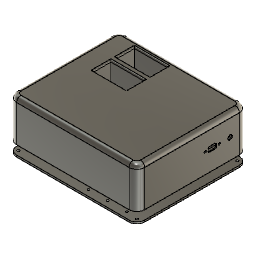
synth case (Autodesk Fusion 360 design; units mm, degrees)
Autodesk Fusion 360 part; units mm, degrees
note: some values were not read from the file. Set by a fixed rule: which sketch regions a step uses.
(part 1 of 2)
sketch "Sketch1" plane through (0, 0, 0) normal (0, 0, 1) x (1, 0, 0) in component "Lid"
  line L0 (6, 0) -> (164, 0) construction
  line L1 (170, 6) -> (170, 139) construction
  line L2 (164, 145) -> (6, 145) construction
  line L3 (0, 139) -> (0, 6) construction
  line L4 (0, 145) -> (10, 145) construction
  line L5 (10, 145) -> (10, 129) construction
  line L6 (10, 129) -> (0, 129) construction
  line L7 (0, 129) -> (0, 145) construction
  line L8 (10, 129) -> (90, 129)
  line L9 (90, 129) -> (90, 126)
  line L10 (90, 126) -> (10, 126)
  line L11 (10, 126) -> (10, 129)
  line L12 (10, 126) -> (10, 96) construction
  line L13 (10, 96) -> (90, 96)
  line L14 (90, 96) -> (90, 93)
  line L15 (90, 93) -> (10, 93)
  line L16 (10, 93) -> (10, 96)
  circle A0 centre (98.5, 65.3144) radius 3.75
  line L17 (24, 66.323) -> (31, 66.323)
  line L18 (33, 64.323) -> (33, 57.323)
  line L19 (31, 55.323) -> (24, 55.323)
  line L20 (22, 57.323) -> (22, 64.323)
  arc A1 (33, 64.323) -> (31, 66.323) centre (31, 64.323) ccw
  arc A2 (31, 55.323) -> (33, 57.323) centre (31, 57.323) ccw
  arc A3 (24, 66.323) -> (22, 64.323) centre (24, 64.323) ccw
  arc A4 (22, 57.323) -> (24, 55.323) centre (24, 57.323) ccw
  line L21 (50, 93) -> (50, 0) construction
  line L22 (98.5, 65.3144) -> (98.5, 57.5144) construction
  circle A5 centre (98.5, 57.5144) radius 1.45
  circle A6 centre (125.5, 65.3144) radius 3.75
  circle A7 centre (125.5, 57.5144) radius 1.45
  circle A8 centre (152.5, 65.3144) radius 3.75
  circle A9 centre (152.5, 57.5144) radius 1.45
  circle A10 centre (98.5, 38.3144) radius 3.75
  circle A11 centre (98.5, 30.5144) radius 1.45
  circle A12 centre (125.5, 38.3144) radius 3.75
  circle A13 centre (125.5, 30.5144) radius 1.45
  circle A14 centre (152.5, 38.3144) radius 3.75
  circle A15 centre (152.5, 30.5144) radius 1.45
  circle A16 centre (98.5, 11.3144) radius 3.75
  circle A17 centre (98.5, 3.5144) radius 1.45
  circle A18 centre (125.5, 11.3144) radius 3.75
  circle A19 centre (125.5, 3.5144) radius 1.45
  circle A20 centre (152.5, 11.3144) radius 3.75
  circle A21 centre (152.5, 3.5144) radius 1.45
  line L23 (170, 38.3144) -> (125.5, 38.3144) construction
  line L24 (97, 139.5) -> (160, 139.5) construction
  line L25 (160, 139.5) -> (160, 115.5) construction
  line L26 (160, 115.5) -> (97, 115.5) construction
  line L27 (97, 115.5) -> (97, 139.5) construction
  line L28 (97, 115.5) -> (160, 139.5) construction
  circle A22 centre (97, 139.5) radius 1.65
  circle A23 centre (160, 139.5) radius 1.65
  circle A24 centre (97, 115.5) radius 1.65
  circle A25 centre (160, 115.5) radius 1.65
  line L29 (113.5, 104.6144) -> (137.5, 104.6144) construction
  line L30 (137.5, 104.6144) -> (137.5, 77.8144) construction
  line L31 (137.5, 77.8144) -> (113.5, 77.8144) construction
  line L32 (113.5, 77.8144) -> (113.5, 104.6144) construction
  circle A26 centre (113.5, 104.6144) radius 1.45
  circle A27 centre (137.5, 104.6144) radius 1.45
  circle A28 centre (113.5, 77.8144) radius 1.45
  circle A29 centre (137.5, 77.8144) radius 1.45
  line L33 (138.5, 101.6644) -> (112.5, 101.6644)
  line L34 (112.5, 101.6644) -> (112.5, 86.6644)
  line L35 (112.5, 86.6644) -> (138.5, 86.6644)
  line L36 (138.5, 86.6644) -> (138.5, 101.6644)
  line L37 (113.5, 103.1644) -> (113.5, 101.6644) construction
  line L38 (113.5, 101.6644) -> (112.5, 101.6644) construction
  arc A30 (170, 139) -> (164, 145) centre (164, 139) ccw construction
  arc A31 (6, 145) -> (0, 139) centre (6, 139) ccw construction
  arc A32 (0, 6) -> (6, 0) centre (6, 6) ccw construction
  arc A33 (164, 0) -> (170, 6) centre (164, 6) ccw construction
  line L39 (125.5, 65.3144) -> (125.5, 77.8144)
  arc A34 (37, 57.323) -> (39, 55.323) centre (39, 57.323) ccw
  line L40 (37, 57.323) -> (37, 64.323)
  arc A35 (39, 66.323) -> (37, 64.323) centre (39, 64.323) ccw
  line L41 (39, 66.323) -> (46, 66.323)
  arc A36 (48, 64.323) -> (46, 66.323) centre (46, 64.323) ccw
  line L42 (48, 64.323) -> (48, 57.323)
  arc A37 (46, 55.323) -> (48, 57.323) centre (46, 57.323) ccw
  line L43 (46, 55.323) -> (39, 55.323)
  arc A38 (52, 57.323) -> (54, 55.323) centre (54, 57.323) ccw
  line L44 (52, 57.323) -> (52, 64.323)
  arc A39 (54, 66.323) -> (52, 64.323) centre (54, 64.323) ccw
  line L45 (54, 66.323) -> (61, 66.323)
  arc A40 (63, 64.323) -> (61, 66.323) centre (61, 64.323) ccw
  line L46 (63, 64.323) -> (63, 57.323)
  arc A41 (61, 55.323) -> (63, 57.323) centre (61, 57.323) ccw
  line L47 (61, 55.323) -> (54, 55.323)
  arc A42 (67, 57.323) -> (69, 55.323) centre (69, 57.323) ccw
  line L48 (67, 57.323) -> (67, 64.323)
  arc A43 (69, 66.323) -> (67, 64.323) centre (69, 64.323) ccw
  line L49 (69, 66.323) -> (76, 66.323)
  arc A44 (78, 64.323) -> (76, 66.323) centre (76, 64.323) ccw
  line L50 (78, 64.323) -> (78, 57.323)
  arc A45 (76, 55.323) -> (78, 57.323) centre (76, 57.323) ccw
  line L51 (76, 55.323) -> (69, 55.323)
  arc A46 (22, 42.323) -> (24, 40.323) centre (24, 42.323) ccw
  line L52 (22, 42.323) -> (22, 49.323)
  arc A47 (24, 51.323) -> (22, 49.323) centre (24, 49.323) ccw
  line L53 (24, 51.323) -> (31, 51.323)
  arc A48 (33, 49.323) -> (31, 51.323) centre (31, 49.323) ccw
  line L54 (33, 49.323) -> (33, 42.323)
  arc A49 (31, 40.323) -> (33, 42.323) centre (31, 42.323) ccw
  line L55 (31, 40.323) -> (24, 40.323)
  arc A50 (37, 42.323) -> (39, 40.323) centre (39, 42.323) ccw
  line L56 (37, 42.323) -> (37, 49.323)
  arc A51 (39, 51.323) -> (37, 49.323) centre (39, 49.323) ccw
  line L57 (39, 51.323) -> (46, 51.323)
  arc A52 (48, 49.323) -> (46, 51.323) centre (46, 49.323) ccw
  line L58 (48, 49.323) -> (48, 42.323)
  arc A53 (46, 40.323) -> (48, 42.323) centre (46, 42.323) ccw
  line L59 (46, 40.323) -> (39, 40.323)
  arc A54 (52, 42.323) -> (54, 40.323) centre (54, 42.323) ccw
  line L60 (52, 42.323) -> (52, 49.323)
  arc A55 (54, 51.323) -> (52, 49.323) centre (54, 49.323) ccw
  line L61 (54, 51.323) -> (61, 51.323)
  arc A56 (63, 49.323) -> (61, 51.323) centre (61, 49.323) ccw
  line L62 (63, 49.323) -> (63, 42.323)
  arc A57 (61, 40.323) -> (63, 42.323) centre (61, 42.323) ccw
  line L63 (61, 40.323) -> (54, 40.323)
  arc A58 (67, 42.323) -> (69, 40.323) centre (69, 42.323) ccw
  line L64 (67, 42.323) -> (67, 49.323)
  arc A59 (69, 51.323) -> (67, 49.323) centre (69, 49.323) ccw
  line L65 (69, 51.323) -> (76, 51.323)
  arc A60 (78, 49.323) -> (76, 51.323) centre (76, 49.323) ccw
  line L66 (78, 49.323) -> (78, 42.323)
  arc A61 (76, 40.323) -> (78, 42.323) centre (76, 42.323) ccw
  line L67 (76, 40.323) -> (69, 40.323)
  arc A62 (22, 27.323) -> (24, 25.323) centre (24, 27.323) ccw
  line L68 (22, 27.323) -> (22, 34.323)
  arc A63 (24, 36.323) -> (22, 34.323) centre (24, 34.323) ccw
  line L69 (24, 36.323) -> (31, 36.323)
  arc A64 (33, 34.323) -> (31, 36.323) centre (31, 34.323) ccw
  line L70 (33, 34.323) -> (33, 27.323)
  arc A65 (31, 25.323) -> (33, 27.323) centre (31, 27.323) ccw
  line L71 (31, 25.323) -> (24, 25.323)
  arc A66 (37, 27.323) -> (39, 25.323) centre (39, 27.323) ccw
  line L72 (37, 27.323) -> (37, 34.323)
  arc A67 (39, 36.323) -> (37, 34.323) centre (39, 34.323) ccw
  line L73 (39, 36.323) -> (46, 36.323)
  arc A68 (48, 34.323) -> (46, 36.323) centre (46, 34.323) ccw
  line L74 (48, 34.323) -> (48, 27.323)
  arc A69 (46, 25.323) -> (48, 27.323) centre (46, 27.323) ccw
  line L75 (46, 25.323) -> (39, 25.323)
  arc A70 (52, 27.323) -> (54, 25.323) centre (54, 27.323) ccw
  line L76 (52, 27.323) -> (52, 34.323)
  arc A71 (54, 36.323) -> (52, 34.323) centre (54, 34.323) ccw
  line L77 (54, 36.323) -> (61, 36.323)
  arc A72 (63, 34.323) -> (61, 36.323) centre (61, 34.323) ccw
  line L78 (63, 34.323) -> (63, 27.323)
  arc A73 (61, 25.323) -> (63, 27.323) centre (61, 27.323) ccw
  line L79 (61, 25.323) -> (54, 25.323)
  arc A74 (67, 27.323) -> (69, 25.323) centre (69, 27.323) ccw
  line L80 (67, 27.323) -> (67, 34.323)
  arc A75 (69, 36.323) -> (67, 34.323) centre (69, 34.323) ccw
  line L81 (69, 36.323) -> (76, 36.323)
  arc A76 (78, 34.323) -> (76, 36.323) centre (76, 34.323) ccw
  line L82 (78, 34.323) -> (78, 27.323)
  arc A77 (76, 25.323) -> (78, 27.323) centre (76, 27.323) ccw
  line L83 (76, 25.323) -> (69, 25.323)
  arc A78 (22, 12.323) -> (24, 10.323) centre (24, 12.323) ccw
  line L84 (22, 12.323) -> (22, 19.323)
  arc A79 (24, 21.323) -> (22, 19.323) centre (24, 19.323) ccw
  line L85 (24, 21.323) -> (31, 21.323)
  arc A80 (33, 19.323) -> (31, 21.323) centre (31, 19.323) ccw
  line L86 (33, 19.323) -> (33, 12.323)
  arc A81 (31, 10.323) -> (33, 12.323) centre (31, 12.323) ccw
  line L87 (31, 10.323) -> (24, 10.323)
  arc A82 (37, 12.323) -> (39, 10.323) centre (39, 12.323) ccw
  line L88 (37, 12.323) -> (37, 19.323)
  arc A83 (39, 21.323) -> (37, 19.323) centre (39, 19.323) ccw
  line L89 (39, 21.323) -> (46, 21.323)
  arc A84 (48, 19.323) -> (46, 21.323) centre (46, 19.323) ccw
  line L90 (48, 19.323) -> (48, 12.323)
  arc A85 (46, 10.323) -> (48, 12.323) centre (46, 12.323) ccw
  line L91 (46, 10.323) -> (39, 10.323)
  arc A86 (52, 12.323) -> (54, 10.323) centre (54, 12.323) ccw
  line L92 (52, 12.323) -> (52, 19.323)
  arc A87 (54, 21.323) -> (52, 19.323) centre (54, 19.323) ccw
  line L93 (54, 21.323) -> (61, 21.323)
  arc A88 (63, 19.323) -> (61, 21.323) centre (61, 19.323) ccw
  line L94 (63, 19.323) -> (63, 12.323)
  arc A89 (61, 10.323) -> (63, 12.323) centre (61, 12.323) ccw
  line L95 (61, 10.323) -> (54, 10.323)
  arc A90 (67, 12.323) -> (69, 10.323) centre (69, 12.323) ccw
  line L96 (67, 12.323) -> (67, 19.323)
  arc A91 (69, 21.323) -> (67, 19.323) centre (69, 19.323) ccw
  line L97 (69, 21.323) -> (76, 21.323)
  arc A92 (78, 19.323) -> (76, 21.323) centre (76, 19.323) ccw
  line L98 (78, 19.323) -> (78, 12.323)
  arc A93 (76, 10.323) -> (78, 12.323) centre (76, 12.323) ccw
  line L99 (76, 10.323) -> (69, 10.323)
  line L100 (57.5, 10.323) -> (57.5, 0) construction
  line L101 (97, 115.5) -> (106, 115.5) construction
  line L102 (106, 115.5) -> (145, 115.5) construction
  line L103 (106, 115.5) -> (106, 139.5)
  line L104 (97, 117.15) -> (145, 117.15)
  line L105 (97, 137.85) -> (145, 137.85)
  line L106 (145, 117.15) -> (106, 137.85) construction
  line L107 (145, 137.85) -> (106, 117.15) construction
  circle A94 centre (125.5, 127.5) radius 6
  circle A95 centre (125.5, 127.5) radius 8
  line L108 (145.4688, 118.0333) -> (106.4688, 138.7333)
  line L109 (144.5312, 116.2667) -> (105.5312, 136.9667)
  line L110 (144.5312, 138.7333) -> (105.5312, 118.0333)
  line L111 (145.4688, 136.9667) -> (106.4688, 116.2667)
  line L112 (145, 137.85) -> (145, 117.15)
  line L113 (90, 127.5) -> (134.3522, 127.5) construction
  line L114 (125.5, 104.6144) -> (125.5, 127.5) construction
  line L115 (-5, 139) -> (-5, 6)
  arc A96 (-5, 6) -> (6, -5) centre (6, 6) ccw
  line L116 (6, -5) -> (164, -5)
  arc A97 (164, -5) -> (175, 6) centre (164, 6) ccw
  line L117 (175, 6) -> (175, 139)
  arc A98 (175, 139) -> (164, 150) centre (164, 139) ccw
  line L118 (164, 150) -> (6, 150)
  arc A99 (6, 150) -> (-5, 139) centre (6, 139) ccw
  circle A100 centre (168.2426, 143.2426) radius 1.65
  circle A101 centre (168.2426, 1.7574) radius 1.65
  circle A102 centre (1.7574, 1.7574) radius 1.65
  circle A103 centre (1.7574, 143.2426) radius 1.65
  line L119 (160, 127.5) -> (170, 127.5) construction
  line L120 (47.4142, 35.7372) -> (52.5858, 40.9087) construction
  line L121 (94.75, 38.323) -> (50, 38.323) construction
  point P0 (170, 0)
  point P1 (22, 66.323)
  point P2 (33, 66.323)
  point P3 (22, 55.323)
  dimension "d1" = 170
  dimension "d2" = 145
  dimension "d3" = 10
  dimension "d4" = 16
  dimension "d5" = 80
  dimension "d6" = 3
  dimension "d7" = 30
  dimension "d8" = 80
  dimension "d9" = 3
  dimension "d10" = 7.5
  dimension "d14" = 11
  dimension "d15" = 11
  dimension "d16" = 2
  dimension "d17" = 2
  dimension "d18" = 2
  dimension "d19" = 2
  dimension "d24" = 7.8
  dimension "d25" = 2.9
  dimension "d28" = 54
  dimension "d29" = -54
  dimension "d31" = 63
  dimension "d32" = 24
  dimension "d33" = 3.3
  dimension "d34" = 3.3
  dimension "d35" = 3.3
  dimension "d36" = 3.3
  dimension "d37" = 24
  dimension "d38" = 26.8
  dimension "d39" = 2.9
  dimension "d40" = 2.9
  dimension "d41" = 2.9
  dimension "d42" = 2.9
  dimension "d43" = 26
  dimension "d44" = 15
  dimension "d45" = 1.5
  dimension "d46" = 1
  dimension "d49" = 6
  dimension "d50" = 6
  dimension "d51" = 6
  dimension "d52" = 6
  dimension "d53" = 12.5
  dimension "d56" = 15
  dimension "d57" = -15
  dimension "d59" = 9
  dimension "d60" = 39
  dimension "d61" = 12
  dimension "d62" = 16
  dimension "d63" = 1
  dimension "d64" = -1
  dimension "d65" = 1
  dimension "d66" = -1
  dimension "d69" = 48
  dimension "d70" = 5
  dimension "d71" = 3.3
  dimension "d72" = 3.3
  dimension "d73" = 3.3
  dimension "d74" = 3.3
  dimension "d81" = 10
  constraint horizontal L0
  constraint vertical L1
  constraint horizontal L2
  constraint vertical L3
  constraint horizontal L4
  constraint vertical L5
  constraint horizontal L6
  constraint vertical L7
  constraint horizontal L8
  constraint vertical L9
  constraint horizontal L10
  constraint vertical L11
  constraint perpendicular L10 L12
  constraint horizontal L13
  constraint vertical L14
  constraint horizontal L15
  constraint vertical L16
  constraint horizontal L17
  constraint vertical L18
  constraint horizontal L19
  constraint vertical L20
  constraint coincident P2 L17
  constraint coincident P2 L18
  constraint tangent L17 A1
  constraint tangent L18 A1
  constraint tangent L18 A2
  constraint tangent L19 A2
  constraint coincident P1 L17
  constraint coincident P1 L20
  constraint tangent L17 A3
  constraint tangent L20 A3
  constraint coincident P3 L19
  constraint coincident P3 L20
  constraint tangent L19 A4
  constraint tangent L20 A4
  constraint midpoint L15 L21.start
  constraint coincident L0 L21.end
  constraint perpendicular L0 L21
  constraint coincident A0.centre L22.start
  constraint vertical L22
  constraint coincident L22.end A5.centre
  constraint coincident L1 L23.start
  constraint coincident A12.centre L23.end
  constraint horizontal L24
  constraint vertical L25
  constraint horizontal L26
  constraint vertical L27
  constraint coincident L24.start L27.end
  constraint coincident L24.end L25.start
  constraint coincident L26.end L27.start
  constraint coincident L25.end L26.start
  constraint horizontal L29
  constraint vertical L30
  constraint horizontal L31
  constraint vertical L32
  constraint coincident L29.start L32.end
  constraint coincident L29.end L30.start
  constraint coincident L31.end L32.start
  constraint coincident L30.end L31.start
  constraint horizontal L33
  constraint vertical L34
  constraint horizontal L35
  constraint vertical L36
  constraint coincident A26 L37.start
  constraint coincident L32 L37.start
  constraint perpendicular L29 L37
  constraint perpendicular L32 L38
  constraint coincident L33.end L34.start
  constraint tangent L1 A30
  constraint tangent L2 A30
  constraint coincident L4.start L2
  constraint coincident L4.start L3
  constraint tangent L2 A31
  constraint tangent L3 A31
  constraint coincident origin L3
  constraint coincident origin L0
  constraint tangent L3 A32
  constraint tangent L0 A32
  constraint coincident P0 L0
  constraint coincident P0 L1
  constraint tangent L0 A33
  constraint tangent L1 A33
  constraint coincident A6.centre L39.start
  constraint vertical L39
  constraint midpoint L31 L39.end
  constraint perpendicular L1 L23
  constraint midpoint L95 L100.start
  constraint coincident L0 L100.end
  constraint perpendicular L0 L100
  constraint parallel L26 L101
  constraint parallel L26 L102
  constraint coincident L24 L103.end
  constraint perpendicular L24 L103
  constraint coincident A24 L104.start
  constraint coincident L27 L104.start
  constraint tangent A24 L104
  constraint coincident A22 L105.start
  constraint coincident L27 L105.start
  constraint tangent A22 L105
  constraint coincident L105 L106.end
  constraint coincident L103 L106.end
  constraint coincident L103 L107.end
  constraint coincident L104 L107.end
  constraint midpoint L106 A94.centre
  constraint concentric A94 A95
  constraint midpoint L9 L113.start
  constraint perpendicular L9 L113
  constraint midpoint L29 L114.start
  constraint coincident L113 A94.centre
  constraint perpendicular L113 L114
  constraint coincident A94.centre A95.centre
  constraint midpoint A30 A100.centre
  constraint midpoint A33 A101.centre
  constraint midpoint A32 A102.centre
  constraint midpoint A31 A103.centre
  constraint midpoint L25 L119.start
  constraint coincident L1 L119.end
  constraint perpendicular L1 L119
  constraint perpendicular L104 L112
  constraint midpoint A68 L120.start
  constraint midpoint A54 L120.end
  constraint coincident A10 L121.start
  constraint coincident L21 L121.end
  constraint perpendicular L21 L121
  constraint midpoint L120 L121.end
  measures "d1" distance of origin P0
  measures "d2" distance of origin L4.start
  measures "d3" distance of L4.start L4.end
  measures "d4" distance of L4.start L6.end
  measures "d5" distance of L5.end L8.end
  measures "d6" distance of L5.end L10.end
  measures "d7" distance of L10.end L12.end
  measures "d8" distance of L12.end L13.end
  measures "d9" distance of L12.end L15.end
  measures "d10" diameter of A0
  measures "d14" distance of P1 P2
  measures "d15" distance of P1 P3
  measures "d16" radius of A1
  measures "d17" radius of A2
  measures "d18" radius of A3
  measures "d19" radius of A4
  measures "d24" distance of A0.centre L22.end
  measures "d25" diameter of A5
  measures "d31" distance of L24.start L24.end
  measures "d32" distance of L24.start L26.end
  measures "d33" diameter of A22
  measures "d34" diameter of A23
  measures "d35" diameter of A24
  measures "d36" diameter of A25
  measures "d37" distance of L29.start L29.end
  measures "d38" distance of L29.start L31.end
  measures "d39" diameter of A26
  measures "d40" diameter of A27
  measures "d41" diameter of A28
  measures "d42" diameter of A29
  measures "d43" distance of L33.start L33.end
  measures "d44" distance of L33.start L35.end
  measures "d45" distance of L37.start L37.end
  measures "d46" distance of L37.end L33.end
  measures "d49" radius of A30
  measures "d50" radius of A31
  measures "d51" radius of A32
  measures "d52" radius of A33
  measures "d53" distance of A6.centre L39.end
  measures "d59" distance of L26.end L101.end
  measures "d60" distance of L101.end L102.end
  measures "d61" diameter of A94
  measures "d62" diameter of A95
  measures "d69" distance of L105.start L105.end
  measures "d71" diameter of A100
  measures "d72" diameter of A101
  measures "d73" diameter of A102
  measures "d74" diameter of A103
  measures "d81" distance of L119.start L119.end
extrude "Extrude4" add sketch "Sketch1" against normal blind 2.5 contours L103 L104 A95 L110 L111 | L103 L105 A95 L108 L109 | A94 A95 L110 L111 | A94 A95 L109 L110 | L104 A95 L108 L109 L112 | A94 A95 L109 L111 | A94 A95 L108 L109 | A94 A95 L108 L109 | A94 A95 L108 L110 | A94 A95 L108 L111 | L105 A95 L110 L111 L112 | A94 A95 L110 L111 | L115 A96 L116 A97 L117 A98 L118 A99 makes body 1 in component "Lid"
extrude "Extrude5" add sketch "Sketch1" against normal blind 0.5 contours A5 | A7 | A9 | A11 | A13 | A15 | A17 | A19 | A21 bodies 1 in component "Lid"
ref_plane "WorkPlane1" through (85, 72.5, 52.5) normal (0, 0, -1) x (-1, 0, 0) in component "bottom"
sketch "Sketch1 (2)" plane through (85, 72.5, 52.5) normal (0, 0, -1) x (1, 0, 0) in component "bottom"
  arc A0 (-24, 51.177) -> (-22, 53.177) centre (-24, 53.177) ccw construction
  line L0 (-24, 51.177) -> (-31, 51.177) construction
  arc A1 (-33, 53.177) -> (-31, 51.177) centre (-31, 53.177) ccw construction
  line L1 (-33, 53.177) -> (-33, 60.177) construction
  arc A2 (-31, 62.177) -> (-33, 60.177) centre (-31, 60.177) ccw construction
  line L2 (-31, 62.177) -> (-24, 62.177) construction
  arc A3 (-22, 60.177) -> (-24, 62.177) centre (-24, 60.177) ccw construction
  line L3 (-22, 60.177) -> (-22, 53.177) construction
  arc A4 (-9, 51.177) -> (-7, 53.177) centre (-9, 53.177) ccw construction
  line L4 (-9, 51.177) -> (-16, 51.177) construction
  arc A5 (-18, 53.177) -> (-16, 51.177) centre (-16, 53.177) ccw construction
  line L5 (-18, 53.177) -> (-18, 60.177) construction
  arc A6 (-16, 62.177) -> (-18, 60.177) centre (-16, 60.177) ccw construction
  line L6 (-16, 62.177) -> (-9, 62.177) construction
  arc A7 (-7, 60.177) -> (-9, 62.177) centre (-9, 60.177) ccw construction
  line L7 (-7, 60.177) -> (-7, 53.177) construction
  arc A8 (-39, 51.177) -> (-37, 53.177) centre (-39, 53.177) ccw construction
  line L8 (-39, 51.177) -> (-46, 51.177) construction
  arc A9 (-48, 53.177) -> (-46, 51.177) centre (-46, 53.177) ccw construction
  line L9 (-48, 53.177) -> (-48, 60.177) construction
  arc A10 (-46, 62.177) -> (-48, 60.177) centre (-46, 60.177) ccw construction
  line L10 (-46, 62.177) -> (-39, 62.177) construction
  arc A11 (-37, 60.177) -> (-39, 62.177) centre (-39, 60.177) ccw construction
  line L11 (-37, 60.177) -> (-37, 53.177) construction
  circle A12 centre (-83.2426, -70.7426) radius 1.65 construction
  arc A13 (-9, 6.177) -> (-7, 8.177) centre (-9, 8.177) ccw construction
  line L12 (-9, 6.177) -> (-16, 6.177) construction
  arc A14 (-18, 8.177) -> (-16, 6.177) centre (-16, 8.177) ccw construction
  line L13 (-18, 8.177) -> (-18, 15.177) construction
  arc A15 (-16, 17.177) -> (-18, 15.177) centre (-16, 15.177) ccw construction
  line L14 (-16, 17.177) -> (-9, 17.177) construction
  arc A16 (-7, 15.177) -> (-9, 17.177) centre (-9, 15.177) ccw construction
  line L15 (-7, 15.177) -> (-7, 8.177) construction
  arc A17 (-54, 21.177) -> (-52, 23.177) centre (-54, 23.177) ccw construction
  line L16 (-54, 21.177) -> (-61, 21.177) construction
  arc A18 (-63, 23.177) -> (-61, 21.177) centre (-61, 23.177) ccw construction
  line L17 (-63, 23.177) -> (-63, 30.177) construction
  arc A19 (-61, 32.177) -> (-63, 30.177) centre (-61, 30.177) ccw construction
  line L18 (-61, 32.177) -> (-54, 32.177) construction
  arc A20 (-52, 30.177) -> (-54, 32.177) centre (-54, 30.177) ccw construction
  line L19 (-52, 30.177) -> (-52, 23.177) construction
  circle A21 centre (28.5, -5.3144) radius 1.45 construction
  circle A22 centre (83.2426, 70.7426) radius 1.65 construction
  arc A23 (-39, 21.177) -> (-37, 23.177) centre (-39, 23.177) ccw construction
  line L20 (-39, 21.177) -> (-46, 21.177) construction
  arc A24 (-48, 23.177) -> (-46, 21.177) centre (-46, 23.177) ccw construction
  line L21 (-48, 23.177) -> (-48, 30.177) construction
  arc A25 (-46, 32.177) -> (-48, 30.177) centre (-46, 30.177) ccw construction
  line L22 (-46, 32.177) -> (-39, 32.177) construction
  arc A26 (-37, 30.177) -> (-39, 32.177) centre (-39, 30.177) ccw construction
  line L23 (-37, 30.177) -> (-37, 23.177) construction
  circle A27 centre (40.5, 7.1856) radius 3.75 construction
  line L24 (53.5, -14.1644) -> (53.5, -29.1644) construction
  line L25 (53.5, -29.1644) -> (27.5, -29.1644) construction
  line L26 (27.5, -29.1644) -> (27.5, -14.1644) construction
  line L27 (27.5, -14.1644) -> (53.5, -14.1644) construction
  circle A28 centre (-83.2426, 70.7426) radius 1.65 construction
  arc A29 (-39, 6.177) -> (-37, 8.177) centre (-39, 8.177) ccw construction
  line L28 (-39, 6.177) -> (-46, 6.177) construction
  arc A30 (-48, 8.177) -> (-46, 6.177) centre (-46, 8.177) ccw construction
  line L29 (-48, 8.177) -> (-48, 15.177) construction
  arc A31 (-46, 17.177) -> (-48, 15.177) centre (-46, 15.177) ccw construction
  line L30 (-46, 17.177) -> (-39, 17.177) construction
  arc A32 (-37, 15.177) -> (-39, 17.177) centre (-39, 15.177) ccw construction
  line L31 (-37, 15.177) -> (-37, 8.177) construction
  arc A33 (-24, 6.177) -> (-22, 8.177) centre (-24, 8.177) ccw construction
  line L32 (-24, 6.177) -> (-31, 6.177) construction
  arc A34 (-33, 8.177) -> (-31, 6.177) centre (-31, 8.177) ccw construction
  line L33 (-33, 8.177) -> (-33, 15.177) construction
  arc A35 (-31, 17.177) -> (-33, 15.177) centre (-31, 15.177) ccw construction
  line L34 (-31, 17.177) -> (-24, 17.177) construction
  arc A36 (-22, 15.177) -> (-24, 17.177) centre (-24, 15.177) ccw construction
  line L35 (-22, 15.177) -> (-22, 8.177) construction
  circle A37 centre (52.5, -5.3144) radius 1.45 construction
  arc A38 (-24, 36.177) -> (-22, 38.177) centre (-24, 38.177) ccw construction
  line L36 (-24, 36.177) -> (-31, 36.177) construction
  arc A39 (-33, 38.177) -> (-31, 36.177) centre (-31, 38.177) ccw construction
  line L37 (-33, 38.177) -> (-33, 45.177) construction
  arc A40 (-31, 47.177) -> (-33, 45.177) centre (-31, 45.177) ccw construction
  line L38 (-31, 47.177) -> (-24, 47.177) construction
  arc A41 (-22, 45.177) -> (-24, 47.177) centre (-24, 45.177) ccw construction
  line L39 (-22, 45.177) -> (-22, 38.177) construction
  arc A42 (-9, 36.177) -> (-7, 38.177) centre (-9, 38.177) ccw construction
  line L40 (-9, 36.177) -> (-16, 36.177) construction
  arc A43 (-18, 38.177) -> (-16, 36.177) centre (-16, 38.177) ccw construction
  line L41 (-18, 38.177) -> (-18, 45.177) construction
  arc A44 (-16, 47.177) -> (-18, 45.177) centre (-16, 45.177) ccw construction
  line L42 (-16, 47.177) -> (-9, 47.177) construction
  arc A45 (-7, 45.177) -> (-9, 47.177) centre (-9, 45.177) ccw construction
  line L43 (-7, 45.177) -> (-7, 38.177) construction
  arc A46 (-54, 51.177) -> (-52, 53.177) centre (-54, 53.177) ccw construction
  line L44 (-54, 51.177) -> (-61, 51.177) construction
  arc A47 (-63, 53.177) -> (-61, 51.177) centre (-61, 53.177) ccw construction
  line L45 (-63, 53.177) -> (-63, 60.177) construction
  arc A48 (-61, 62.177) -> (-63, 60.177) centre (-61, 60.177) ccw construction
  line L46 (-61, 62.177) -> (-54, 62.177) construction
  arc A49 (-52, 60.177) -> (-54, 62.177) centre (-54, 60.177) ccw construction
  line L47 (-52, 60.177) -> (-52, 53.177) construction
  circle A50 centre (52.5, -32.1144) radius 1.45 construction
  arc A51 (-24, 21.177) -> (-22, 23.177) centre (-24, 23.177) ccw construction
  line L48 (-24, 21.177) -> (-31, 21.177) construction
  arc A52 (-33, 23.177) -> (-31, 21.177) centre (-31, 23.177) ccw construction
  line L49 (-33, 23.177) -> (-33, 30.177) construction
  arc A53 (-31, 32.177) -> (-33, 30.177) centre (-31, 30.177) ccw construction
  line L50 (-31, 32.177) -> (-24, 32.177) construction
  arc A54 (-22, 30.177) -> (-24, 32.177) centre (-24, 30.177) ccw construction
  line L51 (-22, 30.177) -> (-22, 23.177) construction
  arc A55 (-9, 21.177) -> (-7, 23.177) centre (-9, 23.177) ccw construction
  line L52 (-9, 21.177) -> (-16, 21.177) construction
  arc A56 (-18, 23.177) -> (-16, 21.177) centre (-16, 23.177) ccw construction
  line L53 (-18, 23.177) -> (-18, 30.177) construction
  arc A57 (-16, 32.177) -> (-18, 30.177) centre (-16, 30.177) ccw construction
  line L54 (-16, 32.177) -> (-9, 32.177) construction
  arc A58 (-7, 30.177) -> (-9, 32.177) centre (-9, 30.177) ccw construction
  line L55 (-7, 30.177) -> (-7, 23.177) construction
  circle A59 centre (83.2426, -70.7426) radius 1.65 construction
  arc A60 (-54, 36.177) -> (-52, 38.177) centre (-54, 38.177) ccw construction
  line L56 (-54, 36.177) -> (-61, 36.177) construction
  arc A61 (-63, 38.177) -> (-61, 36.177) centre (-61, 38.177) ccw construction
  line L57 (-63, 38.177) -> (-63, 45.177) construction
  arc A62 (-61, 47.177) -> (-63, 45.177) centre (-61, 45.177) ccw construction
  line L58 (-61, 47.177) -> (-54, 47.177) construction
  arc A63 (-52, 45.177) -> (-54, 47.177) centre (-54, 45.177) ccw construction
  line L59 (-52, 45.177) -> (-52, 38.177) construction
  circle A64 centre (67.5, 41.9856) radius 1.45 construction
  circle A65 centre (13.5, 61.1856) radius 3.75 construction
  circle A66 centre (40.5, 41.9856) radius 1.45 construction
  circle A67 centre (13.5, 68.9856) radius 1.45 construction
  line L60 (33.0203, -57.8379) -> (21, -64.2179) construction
  line L61 (21, -64.2179) -> (21, -45.7821) construction
  line L62 (21, -45.7821) -> (33.0203, -52.1621) construction
  arc A68 (33.0203, -52.1621) -> (33.0203, -57.8379) centre (40.5, -55) ccw construction
  circle A69 centre (12, -67) radius 1.65 construction
  line L63 (33.9579, -50.3955) -> (23.133, -44.65) construction
  line L64 (23.133, -44.65) -> (57.867, -44.65) construction
  line L65 (57.867, -44.65) -> (47.0421, -50.3955) construction
  arc A70 (47.0421, -50.3955) -> (33.9579, -50.3955) centre (40.5, -55) ccw construction
  circle A71 centre (12, -43) radius 1.65 construction
  line L66 (23.133, -65.35) -> (33.9579, -59.6045) construction
  arc A72 (33.9579, -59.6045) -> (47.0421, -59.6045) centre (40.5, -55) ccw construction
  line L67 (47.0421, -59.6045) -> (57.867, -65.35) construction
  line L68 (57.867, -65.35) -> (23.133, -65.35) construction
  circle A73 centre (67.5, 34.1856) radius 3.75 construction
  line L69 (60, -45.7821) -> (60, -64.2179) construction
  line L70 (60, -64.2179) -> (47.9797, -57.8379) construction
  arc A74 (47.9797, -57.8379) -> (47.9797, -52.1621) centre (40.5, -55) ccw construction
  line L71 (47.9797, -52.1621) -> (60, -45.7821) construction
  circle A75 centre (40.5, -55) radius 6 construction
  circle A76 centre (13.5, 14.9856) radius 1.45 construction
  circle A77 centre (40.5, 14.9856) radius 1.45 construction
  circle A78 centre (67.5, 68.9856) radius 1.45 construction
  circle A79 centre (67.5, 7.1856) radius 3.75 construction
  circle A80 centre (67.5, 14.9856) radius 1.45 construction
  circle A81 centre (13.5, 34.1856) radius 3.75 construction
  circle A82 centre (13.5, 41.9856) radius 1.45 construction
  circle A83 centre (40.5, 34.1856) radius 3.75 construction
  circle A84 centre (40.5, 61.1856) radius 3.75 construction
  circle A85 centre (67.5, 61.1856) radius 3.75 construction
  circle A86 centre (40.5, 68.9856) radius 1.45 construction
  line L72 (-75, -53.5) -> (5, -53.5) construction
  line L73 (5, -53.5) -> (5, -56.5) construction
  line L74 (5, -56.5) -> (-75, -56.5) construction
  line L75 (-75, -56.5) -> (-75, -53.5) construction
  arc A87 (-63, 8.177) -> (-61, 6.177) centre (-61, 8.177) ccw construction
  line L76 (-63, 8.177) -> (-63, 15.177) construction
  arc A88 (-61, 17.177) -> (-63, 15.177) centre (-61, 15.177) ccw construction
  line L77 (-61, 17.177) -> (-54, 17.177) construction
  arc A89 (-52, 15.177) -> (-54, 17.177) centre (-54, 15.177) ccw construction
  line L78 (-52, 15.177) -> (-52, 8.177) construction
  arc A90 (-54, 6.177) -> (-52, 8.177) centre (-54, 8.177) ccw construction
  line L79 (-54, 6.177) -> (-61, 6.177) construction
  circle A91 centre (13.5, 7.1856) radius 3.75 construction
  line L80 (-75, -20.5) -> (5, -20.5) construction
  line L81 (5, -20.5) -> (5, -23.5) construction
  line L82 (5, -23.5) -> (-75, -23.5) construction
  line L83 (-75, -23.5) -> (-75, -20.5) construction
  arc A92 (-39, 36.177) -> (-37, 38.177) centre (-39, 38.177) ccw construction
  line L84 (-39, 36.177) -> (-46, 36.177) construction
  arc A93 (-48, 38.177) -> (-46, 36.177) centre (-46, 38.177) ccw construction
  line L85 (-48, 38.177) -> (-48, 45.177) construction
  arc A94 (-46, 47.177) -> (-48, 45.177) centre (-46, 45.177) ccw construction
  line L86 (-46, 47.177) -> (-39, 47.177) construction
  arc A95 (-37, 45.177) -> (-39, 47.177) centre (-39, 45.177) ccw construction
  line L87 (-37, 45.177) -> (-37, 38.177) construction
  circle A96 centre (28.5, -32.1144) radius 1.45 construction
  circle A97 centre (75, -43) radius 1.65 construction
  circle A98 centre (75, -67) radius 1.65 construction
  arc A99 (-90, -66.5) -> (-79, -77.5) centre (-79, -66.5) ccw
  line L88 (-79, -77.5) -> (79, -77.5)
  arc A100 (79, -77.5) -> (90, -66.5) centre (79, -66.5) ccw
  line L89 (90, -66.5) -> (90, 66.5)
  arc A101 (90, 66.5) -> (79, 77.5) centre (79, 66.5) ccw
  line L90 (79, 77.5) -> (-79, 77.5)
  arc A102 (-79, 77.5) -> (-90, 66.5) centre (-79, 66.5) ccw
  line L91 (-90, 66.5) -> (-90, -66.5)
  line L92 (-37.5858, 36.7628) -> (-32.4142, 31.5913) construction
  line L93 (-65.2, 3.977) -> (-4.8, 3.977)
  line L94 (-4.8, 3.977) -> (-4.8, 64.377)
  line L95 (-4.8, 64.377) -> (-65.2, 64.377)
  line L96 (-65.2, 64.377) -> (-65.2, 3.977)
  line L97 (-65.2, 3.977) -> (-4.8, 64.377) construction
  line L98 (-2.8, 66.377) -> (-67.2, 66.377)
  line L99 (-67.2, 66.377) -> (-67.2, 1.977)
  line L100 (-67.2, 1.977) -> (-2.8, 1.977)
  line L101 (-2.8, 1.977) -> (-2.8, 66.377)
  line L102 (-67.2, 34.177) -> (-60.2, 34.177)
  line L103 (-60.2, 34.177) -> (-60.2, 26.377)
  line L104 (-60.2, 26.377) -> (-67.2, 26.377)
  line L105 (-67.2, 26.377) -> (-67.2, 34.177)
  line L106 (-60.2, 34.177) -> (-65.2, 34.177)
  line L107 (-65.2, 34.177) -> (-65.2, 41.977)
  line L108 (-65.2, 41.977) -> (-60.2, 41.977)
  line L109 (-60.2, 41.977) -> (-60.2, 34.177)
  line L110 (-35, 1.977) -> (-27.2, 1.977)
  line L111 (-27.2, 1.977) -> (-27.2, 8.977)
  line L112 (-27.2, 8.977) -> (-35, 8.977)
  line L113 (-35, 8.977) -> (-35, 1.977)
  line L114 (-35, 1.977) -> (-42.8, 1.977)
  line L115 (-42.8, 1.977) -> (-42.8, 8.977)
  line L116 (-42.8, 8.977) -> (-35, 8.977)
  line L117 (-35, 8.977) -> (-35, 1.977)
  line L118 (-2.8, 34.177) -> (-9.8, 34.177)
  line L119 (-9.8, 34.177) -> (-9.8, 26.377)
  line L120 (-9.8, 26.377) -> (-2.8, 26.377)
  line L121 (-2.8, 26.377) -> (-2.8, 34.177)
  line L122 (-2.8, 34.177) -> (-9.8, 34.177)
  line L123 (-9.8, 34.177) -> (-9.8, 41.977)
  line L124 (-9.8, 41.977) -> (-2.8, 41.977)
  line L125 (-2.8, 41.977) -> (-2.8, 34.177)
  line L126 (-35, 66.377) -> (-42.8, 66.377)
  line L127 (-42.8, 66.377) -> (-42.8, 59.377)
  line L128 (-42.8, 59.377) -> (-35, 59.377)
  line L129 (-35, 59.377) -> (-35, 66.377)
  line L130 (-35, 66.377) -> (-27.2, 66.377)
  line L131 (-27.2, 66.377) -> (-27.2, 59.377)
  line L132 (-27.2, 59.377) -> (-35, 59.377)
  line L133 (-35, 59.377) -> (-35, 66.377)
  line L134 (-60.2, 41.977) -> (-60.2, 64.377)
  line L135 (-42.8, 59.377) -> (-65.2, 59.377)
  line L136 (-60.2, 26.377) -> (-60.2, 3.977)
  line L137 (-42.8, 8.977) -> (-65.2, 8.977)
  line L138 (-27.2, 8.977) -> (-4.8, 8.977)
  line L139 (-9.8, 26.377) -> (-9.8, 3.977)
  line L140 (-9.8, 41.977) -> (-9.8, 64.377)
  line L141 (-27.2, 59.377) -> (-9.8, 59.377)
  line L142 (-15.95, -13.75) -> (-54.05, -13.75) construction
  line L143 (-54.05, -13.75) -> (-54.05, -30.25) construction
  line L144 (-54.05, -30.25) -> (-15.95, -30.25) construction
  line L145 (-15.95, -30.25) -> (-15.95, -13.75) construction
  line L146 (-54.05, -46.75) -> (-54.05, -63.25) construction
  line L147 (-54.05, -63.25) -> (-15.95, -63.25) construction
  line L148 (-15.95, -46.75) -> (-54.05, -46.75) construction
  line L149 (-15.95, -63.25) -> (-15.95, -46.75) construction
  line L150 (5, -20.5) -> (-75, -23.5) construction
  line L151 (-75, -56.5) -> (5, -53.5) construction
  line L152 (-15.95, -30.25) -> (-54.05, -13.75) construction
  line L153 (-54.05, -46.75) -> (-15.95, -63.25) construction
  circle A103 centre (-15.95, -13.75) radius 1.4
  circle A104 centre (-15.95, -30.25) radius 1.4
  circle A105 centre (-54.05, -13.75) radius 1.4
  circle A106 centre (-15.95, -46.75) radius 1.4
  circle A107 centre (-15.95, -63.25) radius 1.4
  circle A108 centre (-54.05, -46.75) radius 1.4
  circle A109 centre (-54.05, -63.25) radius 1.4
  circle A110 centre (-15.95, -13.75) radius 3.5
  circle A111 centre (-15.95, -30.25) radius 3.5
  circle A112 centre (-54.05, -13.75) radius 3.5
  circle A113 centre (-54.05, -30.25) radius 1.4
  circle A114 centre (-54.05, -30.25) radius 3.5
  circle A115 centre (-15.95, -46.75) radius 3.5
  circle A116 centre (-15.95, -63.25) radius 3.5
  circle A117 centre (-54.05, -46.75) radius 3.5
  circle A118 centre (-54.05, -63.25) radius 3.5
  circle A119 centre (-54.05, -13.75) radius 2.5
  circle A120 centre (-15.95, -13.75) radius 2.5
  circle A121 centre (-54.05, -30.25) radius 2.5
  circle A122 centre (-15.95, -30.25) radius 2.5
  circle A123 centre (-15.95, -46.75) radius 2.5
  circle A124 centre (-15.95, -63.25) radius 2.5
  circle A125 centre (-54.05, -46.75) radius 2.5
  circle A126 centre (-54.05, -63.25) radius 2.5
  line L154 (-60, -41) -> (-10, -41)
  line L155 (-10, -41) -> (-10, -69)
  line L156 (-10, -69) -> (-60, -69)
  line L157 (-60, -69) -> (-60, -41)
  line L158 (-60, -69) -> (-10, -41) construction
  line L159 (-60, -8) -> (-10, -8)
  line L160 (-60, -36) -> (-60, -8)
  line L161 (-60, -36) -> (-10, -8) construction
  line L162 (-10, -36) -> (-60, -36)
  line L163 (-10, -8) -> (-10, -36)
  line L164 (-12, -34) -> (-58, -34)
  line L165 (-58, -34) -> (-58, -10)
  line L166 (-58, -10) -> (-12, -10)
  line L167 (-12, -10) -> (-12, -34)
  line L168 (-58, -67) -> (-58, -43)
  line L169 (-58, -43) -> (-12, -43)
  line L170 (-12, -43) -> (-12, -67)
  line L171 (-12, -67) -> (-58, -67)
  line L172 (-65.2, 41.977) -> (-67.2, 41.977)
  circle A127 centre (-83.2426, -70.7426) radius 2.2
  circle A128 centre (-83.2426, -70.7426) radius 5
  circle A129 centre (83.2426, -70.7426) radius 2.2
  circle A130 centre (83.2426, 70.7426) radius 2.2
  circle A131 centre (-83.2426, 70.7426) radius 2.2
  circle A132 centre (-83.2426, 70.7426) radius 5
  circle A133 centre (83.2426, 70.7426) radius 5
  circle A134 centre (83.2426, -70.7426) radius 5
  arc A135 (85, 66.5) -> (79, 72.5) centre (79, 66.5) ccw
  line L173 (79, 72.5) -> (-79, 72.5)
  arc A136 (-79, 72.5) -> (-85, 66.5) centre (-79, 66.5) ccw
  line L174 (-85, 66.5) -> (-85, -66.5)
  arc A137 (-85, -66.5) -> (-79, -72.5) centre (-79, -66.5) ccw
  line L175 (-79, -72.5) -> (79, -72.5)
  arc A138 (79, -72.5) -> (85, -66.5) centre (79, -66.5) ccw
  line L176 (85, -66.5) -> (85, 66.5)
  dimension "d85" = 60.4
  dimension "d86" = 60.4
  dimension "d87" = 2
  dimension "d88" = 7
  dimension "d89" = 7.8
  dimension "d90" = 7.8
  dimension "d91" = 7.8
  dimension "d92" = 7
  dimension "d93" = 7.8
  dimension "d94" = 7
  dimension "d95" = 7
  dimension "d96" = 7.8
  dimension "d97" = 7
  dimension "d98" = 7.8
  dimension "d99" = 7.8
  dimension "d100" = 7
  dimension "d101" = 7.8
  dimension "d102" = 7
  dimension "d103" = 38.1
  dimension "d104" = 16.5
  dimension "d105" = 38.1
  dimension "d106" = 16.5
  dimension "d107" = 2.8
  dimension "d108" = 2.8
  dimension "d109" = 2.8
  dimension "d110" = 2.8
  dimension "d111" = 2.8
  dimension "d112" = 2.8
  dimension "d113" = 2.8
  dimension "d114" = 7
  dimension "d115" = 7
  dimension "d116" = 7
  dimension "d117" = 2.8
  dimension "d118" = 7
  dimension "d119" = 7
  dimension "d120" = 7
  dimension "d121" = 7
  dimension "d122" = 7
  dimension "d123" = 5
  dimension "d124" = 5
  dimension "d125" = 5
  dimension "d126" = 5
  dimension "d127" = 5
  dimension "d128" = 5
  dimension "d129" = 5
  dimension "d130" = 5
  dimension "d131" = 50
  dimension "d132" = 28
  dimension "d133" = 50
  dimension "d134" = 28
  dimension "d135" = 2
  dimension "d140" = 4.4
  dimension "d141" = 4.4
  dimension "d142" = 4.4
  dimension "d143" = 4.4
  dimension "d144" = -5
  constraint midpoint A92 L92.start
  constraint midpoint A53 L92.end
  constraint horizontal L93
  constraint vertical L94
  constraint horizontal L95
  constraint vertical L96
  constraint midpoint L92 L97
  constraint horizontal L102
  constraint vertical L103
  constraint horizontal L104
  constraint vertical L105
  constraint midpoint L99 L102.start
  constraint horizontal L106
  constraint vertical L107
  constraint horizontal L108
  constraint vertical L109
  constraint horizontal L110
  constraint vertical L111
  constraint horizontal L112
  constraint vertical L113
  constraint midpoint L100 L110.start
  constraint horizontal L114
  constraint vertical L115
  constraint horizontal L116
  constraint vertical L117
  constraint horizontal L118
  constraint vertical L119
  constraint horizontal L120
  constraint vertical L121
  constraint midpoint L101 L118.start
  constraint horizontal L122
  constraint vertical L123
  constraint horizontal L124
  constraint vertical L125
  constraint horizontal L126
  constraint vertical L127
  constraint horizontal L128
  constraint vertical L129
  constraint midpoint L98 L126.start
  constraint horizontal L130
  constraint vertical L131
  constraint horizontal L132
  constraint vertical L133
  constraint coincident L95 L134.end
  constraint perpendicular L95 L134
  constraint coincident L96 L135.end
  constraint perpendicular L96 L135
  constraint coincident L93 L136.end
  constraint perpendicular L93 L136
  constraint coincident L96 L137.end
  constraint perpendicular L96 L137
  constraint coincident L94 L138.end
  constraint perpendicular L94 L138
  constraint coincident L93 L139.end
  constraint perpendicular L93 L139
  constraint coincident L95 L140.end
  constraint perpendicular L95 L140
  constraint coincident L140 L141.end
  constraint coincident L97 L141.end
  constraint horizontal L142
  constraint vertical L143
  constraint horizontal L144
  constraint vertical L145
  constraint horizontal L148
  constraint vertical L146
  constraint horizontal L147
  constraint vertical L149
  constraint coincident L80.end L81.start
  constraint coincident L82.end L83.start
  constraint coincident L74.end L75.start
  constraint coincident L72.end L73.start
  constraint midpoint L151 L153
  constraint midpoint L150 L152
  constraint coincident L142.start L145.end
  constraint coincident L144.end L145.start
  constraint coincident L142.end L143.start
  constraint coincident L148.start L149.end
  constraint coincident L147.end L149.start
  constraint coincident L146.start L148.end
  constraint coincident L146.end L147.start
  constraint concentric A103 A110
  constraint concentric A104 A111
  constraint concentric A105 A112
  constraint coincident L143.end L144.start
  constraint concentric A113 A114
  constraint concentric A106 A115
  constraint concentric A107 A116
  constraint concentric A108 A117
  constraint concentric A109 A118
  constraint concentric A112 A119
  constraint concentric A110 A120
  constraint concentric A114 A121
  constraint concentric A104 A122
  constraint concentric A106 A123
  constraint concentric A107 A124
  constraint concentric A117 A125
  constraint concentric A118 A126
  constraint horizontal L154
  constraint vertical L155
  constraint horizontal L156
  constraint vertical L157
  constraint horizontal L159
  constraint vertical L163
  constraint horizontal L162
  constraint vertical L160
  constraint midpoint L152 L161
  constraint midpoint L153 L158
  constraint coincident L99 L172.end
  constraint perpendicular L99 L172
  constraint concentric A12 A127
  constraint concentric A127 A128
  constraint tangent A99 A128
  constraint concentric A59 A129
  constraint concentric A22 A130
  constraint concentric A28 A131
  constraint concentric A28 A132
  constraint tangent A102 A132
  constraint concentric A22 A133
  constraint tangent A101 A133
  constraint concentric A59 A134
  constraint tangent A100 A134
  measures "d85" distance of L93.start L93.end
  measures "d86" distance of L93.start L95.end
  measures "d88" distance of L102.start L102.end
  measures "d89" distance of L102.start L104.end
  measures "d90" distance of L102.end L108.end
  measures "d91" distance of L110.start L110.end
  measures "d92" distance of L110.start L112.end
  measures "d93" distance of L110.start L114.end
  measures "d94" distance of L110.start L112.end
  measures "d95" distance of L118.start L118.end
  measures "d96" distance of L118.start L120.end
  measures "d97" distance of L118.start L118.end
  measures "d98" distance of L118.start L124.end
  measures "d99" distance of L126.start L126.end
  measures "d100" distance of L126.start L128.end
  measures "d101" distance of L126.start L130.end
  measures "d102" distance of L126.start L128.end
  measures "d103" distance of L142.start L142.end
  measures "d104" distance of L142.start L144.end
  measures "d105" distance of L146.start L148.start
  measures "d106" distance of L147.end L148.start
  measures "d107" diameter of A103
  measures "d108" diameter of A104
  measures "d109" diameter of A105
  measures "d110" diameter of A106
  measures "d111" diameter of A107
  measures "d112" diameter of A108
  measures "d113" diameter of A109
  measures "d114" diameter of A110
  measures "d115" diameter of A111
  measures "d116" diameter of A112
  measures "d117" diameter of A113
  measures "d118" diameter of A114
  measures "d119" diameter of A115
  measures "d120" diameter of A116
  measures "d121" diameter of A117
  measures "d122" diameter of A118
  measures "d123" diameter of A119
  measures "d124" diameter of A120
  measures "d125" diameter of A121
  measures "d126" diameter of A122
  measures "d127" diameter of A123
  measures "d128" diameter of A124
  measures "d129" diameter of A125
  measures "d130" diameter of A126
  measures "d131" distance of L154.start L154.end
  measures "d132" distance of L154.start L156.end
  measures "d133" distance of L159.start L159.end
  measures "d134" distance of L159.start L160.start
  measures "d140" diameter of A127
  measures "d141" diameter of A129
  measures "d142" diameter of A130
  measures "d143" diameter of A131
move_body "Move1" bodies 1 to x (1, 0, 0) y (0, 1, 0) z (0, 0, 1) at (0, 0, -15) in component "Lid"
extrude "Extrude1" add sketch "Sketch1 (2)" along normal blind 50 separate body contours L93 L96 L136 L137 | L93 L96 L99 L100 L104 L115 | L93 L115 L136 L137 | L96 L104 L136 L137 | L93 L111 L138 L139 | L93 L94 L100 L101 L111 L120 | L95 L96 L98 L99 L127 L172 | L96 L108 L134 L135 | L93 L94 L138 L139 | L95 L96 L134 L135 | L94 L120 L138 L139 | L95 L127 L134 L135 | L94 L95 L124 L140 | L94 L95 L98 L101 L124 L131 | L95 L131 L140 L141 makes body 2 at (82.2, 22.3896, 19.1667) makes body 3 at (65.9333, 70.523, 19.1667) makes body 4 at (17.8, 14.2563, 19.1667) makes body 5 at (17.8, 54.2563, 35.8333) in component "bottom"
sketch "Sketch2" plane through (0, 0, 2.5) normal (0, 0, -1) x (1, 0, 0) in component "bottom"
  line L0 (57.8, -70.523) -> (82.2, -70.523)
  line L1 (82.2, -70.523) -> (82.2, -46.123)
  line L2 (82.2, -46.123) -> (75.2, -46.123)
  line L3 (75.2, -46.123) -> (75.2, -63.523)
  line L4 (75.2, -63.523) -> (57.8, -63.523)
  line L5 (57.8, -63.523) -> (57.8, -70.523)
  line L6 (80.2, -68.523) -> (80.2, -8.123)
  line L7 (19.8, -68.523) -> (80.2, -68.523)
  line L8 (19.8, -8.123) -> (19.8, -68.523)
  line L9 (80.2, -8.123) -> (19.8, -8.123)
  line L10 (82.2, -70.523) -> (82.2, -6.123)
  line L11 (82.2, -6.123) -> (17.8, -6.123)
  line L12 (17.8, -70.523) -> (82.2, -70.523)
  line L13 (17.8, -6.123) -> (17.8, -70.523)
  line L14 (75.2, -46.123) -> (82.2, -46.123)
  line L15 (75.2, -30.523) -> (82.2, -30.523)
  line L16 (57.8, -70.523) -> (57.8, -63.523)
  line L17 (42.2, -70.523) -> (42.2, -63.523)
  line L18 (24.8, -46.123) -> (17.8, -46.123)
  line L19 (19.8, -30.523) -> (17.8, -30.523)
  line L20 (19.8, -30.523) -> (24.8, -30.523)
  line L21 (57.8, -6.123) -> (57.8, -13.123)
  line L22 (42.2, -6.123) -> (42.2, -13.123)
extrude "Extrude2" add sketch "Sketch2" along normal blind 4 contours L0 L1 L2 L5 L6 L7 L10 L12 L14 L16 | L7 L8 L12 L13 L17 L18 | L6 L9 L10 L11 L15 L21 | L8 L9 L11 L13 L19 L22 bodies 2 3 4 5 in component "bottom"
extrude "Extrude4'" add sketch "Sketch1 (2)" along normal blind 49 separate body contours A127 A137 | A127 A137 | A131 A136 | A131 A136 | A129 A138 | A129 A138 | A130 A135 | A130 A135 makes body 6 at (168.2975, -0.442, 36.1667) makes body 7 at (168.2975, 141.0433, 36.1667) makes body 8 at (3.9546, 1.867, 36.1667) makes body 9 at (0.0721, 144.6568, 36.1667) in component "bottom"
extrude "Extrude3" add sketch "Sketch1 (2)" along normal blind 55 separate body contours A99 A102 L91 A128 A132 L174 | A99 L88 A100 A128 A134 L175 | A127 A128 L174 A137 L175 | A127 A128 L174 A137 L175 | A101 L90 A102 A132 A133 L173 | A131 A132 L173 A136 L174 | A131 A132 L173 A136 L174 | A129 A134 L175 A138 L176 | A129 A134 L175 A138 L176 | A100 L89 A101 A133 A134 L176 | A130 A133 A135 L173 L176 | A130 A133 A135 L173 L176 makes body 10 in component "bottom"
extrude "Extrude5'" add sketch "Sketch1 (2)" along normal blind 35 separate body contours L154 L155 L156 L157 | L159 L160 L162 L163 makes body 11 at (41.6667, 80.5, 40.8333) makes body 12 at (41.6667, 113.5, 40.8333) in component "bottom"
sketch "Sketch3" plane through (0, 0, 17.5) normal (0, 0, -1) x (1, 0, 0) in component "bottom"
  line L0 (27, -82.5) -> (73, -82.5)
  line L1 (73, -82.5) -> (73, -106.5)
  line L2 (73, -106.5) -> (27, -106.5)
  line L3 (27, -106.5) -> (27, -82.5)
  line L4 (75, -80.5) -> (25, -80.5)
  line L5 (25, -80.5) -> (25, -108.5)
  line L6 (25, -108.5) -> (75, -108.5)
  line L7 (75, -108.5) -> (75, -80.5)
  circle A0 centre (30.95, -86.25) radius 2.5
  circle A1 centre (30.95, -86.25) radius 1.4
  circle A2 centre (30.95, -102.75) radius 2.5
  circle A3 centre (30.95, -102.75) radius 1.4
  circle A4 centre (69.05, -102.75) radius 2.5
  circle A5 centre (69.05, -102.75) radius 1.4
  circle A6 centre (69.05, -86.25) radius 2.5
  circle A7 centre (69.05, -86.25) radius 1.4
extrude "Extrude6" add sketch "Sketch3" against normal blind 7 contours L0 L1 L2 L3 bodies 11 in component "bottom"